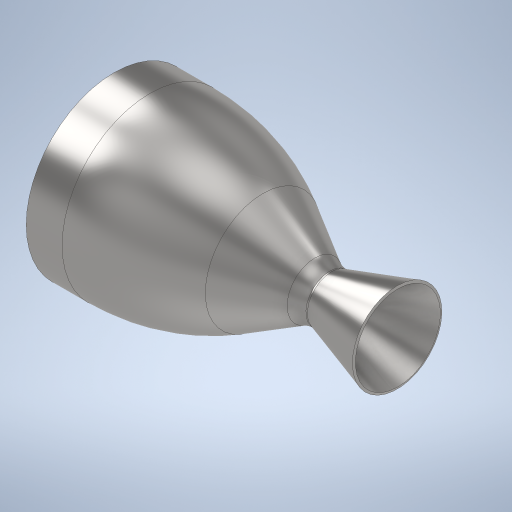
# Autodesk Inventor part: inner wall
Saved by Autodesk Inventor 2023 (Build 270158000, 158)
## iProperties
Created: 2022-07-20
Part Number: inner wall
Material: Stainless Steel
Document SubType Name: Modeling
Designer: station
Density: 8 g/cm^3
Appearance: Semi-Polished
Author: station
Autodesk Inventor part; units mm, degrees
ref_plane "YZ Plane" through (0, 0, 0) normal (1, 0, 0) x (0, 1, 0)
ref_plane "XZ Plane" through (0, 0, 0) normal (0, 1, 0) x (-1, 0, 0)
ref_plane "XY Plane" through (0, 0, 0) normal (0, 0, 1) x (1, 0, 0)
sketch "Sketch1" plane through (0, 0, 0) normal (0, 0, 1) x (1, 0, 0)
  line L0 (123.3912, 50.0622) -> (166.724, 25.044)
  arc A0 (123.3912, 50.0622) -> (30.0219, 75.0805) centre (30.0219, -111.6581) ccw
  arc A1 (166.724, 25.044) -> (180.1312, 21.4516) centre (180.1312, 48.266) ccw
  arc A2 (180.1312, 21.4516) -> (182.1847, 21.7676) centre (180.1312, 28.2803) ccw
  line L1 (0, 75.0805) -> (30.0219, 75.0805)
  line L2 (0, 3.5755) -> (0, 203.5755) construction
  line L3 (0, 3.5755) -> (319.1694, 3.5755)
  line L4 (0, 77.0805) -> (30.0219, 77.0805)
  arc A3 (124.3912, 51.7943) -> (30.0219, 77.0805) centre (30.0219, -111.6581) ccw
  line L5 (124.3912, 51.7943) -> (167.724, 26.7761)
  arc A4 (167.724, 26.7761) -> (180.1312, 23.4516) centre (180.1312, 48.266) ccw
  arc A5 (180.1312, 23.4516) -> (181.5842, 23.6753) centre (180.1312, 28.2803) ccw
  line L6 (0, 77.0805) -> (0, 75.0805)
  line L7 (182.1847, 21.7676) -> (237.115, 39.0871)
  line L8 (236.5136, 40.9945) -> (181.5833, 23.6751)
  arc A6 (180.1312, 23.4516) -> (181.5833, 23.6751) centre (180.1312, 28.2803) ccw
  line L9 (236.5136, 40.9945) -> (237.115, 39.0871)
  point P0 (181.5833, 23.6751)
  point P1 (123.3912, 50.0622)
  point P2 (166.724, 25.044)
  point P3 (181.5842, 23.6753)
  point P4 (30.0219, 75.0805)
  dimension "d51" = 200
  dimension "d52" = 30.0219
  dimension "d53" = 186.7386
  dimension "d54" = 0
  dimension "d55" = 0
  dimension "d56" = 0
  dimension "d74" = 71.505
  dimension "d75" = 2
  dimension "d76" = 2
  dimension "d77" = 2
  dimension "d78" = 2
  dimension "d80" = 2
  dimension "d82" = 17.5
  dimension "d83" = 54.9303
  dimension "d84" = 2
  constraints: 20 end point, 14 point on circle, 7 centre point, 2 parallel, 1 horizontal, 1 perpendicular, 1 tangent, 1 other
  measures "d51" distance of L2.start L2.end
  measures "d52" distance of L1.start L1.end
  measures "d53" radius of A0
  measures "d54" distance from line of L1.start L2
  measures "d55" distance of A0.end L1.end
  measures "d56" distance of L0.start A0.start
  measures "d74" distance between parallel lines of L3 L1
  measures "d75" distance between parallel lines of L1 L4
  measures "d76" radial gap between concentric circles of A0 A3
  measures "d77" distance between parallel lines of L0 L5
  measures "d78" radial gap between concentric circles of A1 A4
  measures "d80" radial gap between concentric circles of A2 A5
  measures "d82" angle of L3 L7
  measures "d83" horizontal distance of L7.start L7.end
  measures "d84" distance between parallel lines of L7 L8
revolve "Revolution2" add sketch "Sketch1" angle 360 about axis through (0, 3.5755, 0) along (1, 0, 0)
body "Solid2"
